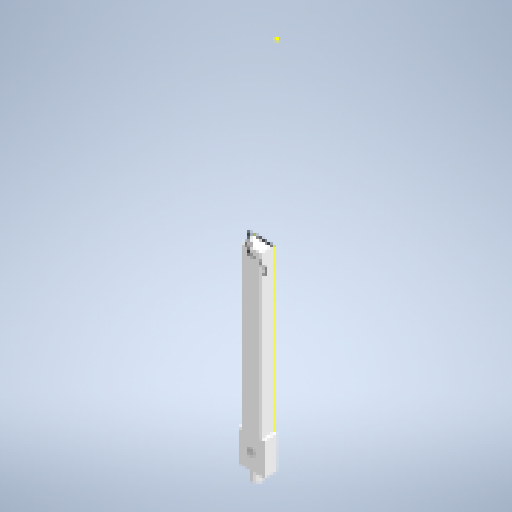
# Autodesk Inventor part: SchubstangeA
Saved by Autodesk Inventor 2025 (Build 290162010, 162A)
## iProperties
Created: 2024-11-26
Part Number: SchubstangeA
Material: PC/ABS-Kunststoff, 3DDruck, PLA
Document SubType Name: Modeling
Designer: Admin
Density: 1.1 g/cm^3
Appearance: Glatt - Weiß(2)
Author: Admin
Autodesk Inventor part; units mm, degrees
ref_plane "YZ Plane" through (0, 0, 0) normal (1, 0, 0) x (0, 1, 0)
ref_plane "XZ Plane" through (0, 0, 0) normal (0, 1, 0) x (-1, 0, 0)
ref_plane "XY Plane" through (0, 0, 0) normal (0, 0, 1) x (1, 0, 0)
sketch "Skizze1" plane through (0, 0, 0) normal (0, 1, 0) x (-1, 0, 0)
  line L0 (6.8592, -116.2444) -> (0.8592, -116.2444)
  line L1 (0.8592, -116.2444) -> (0.8592, -56.2444)
  line L2 (6.8592, -56.2444) -> (6.8592, -116.2444)
  line L3 (7.8592, -116.2444) -> (-0.1408, -116.2444)
  line L4 (-0.1408, -116.2444) -> (-0.1408, -106.2444)
  line L5 (-0.1408, -106.2444) -> (7.8592, -106.2444)
  line L6 (7.8592, -106.2444) -> (7.8592, -116.2444)
  line L7 (3.8592, 157.3916) -> (3.8592, -262.6084)
  line L8 (6.8592, -56.2444) -> (0.8592, -56.2444)
  line L9 (0.8592, -56.2444) -> (-2.1408, -56.2444)
  line L10 (-2.1408, -56.2444) -> (-2.1408, -66.2444)
  line L11 (-2.1408, -66.2444) -> (0.8592, -66.2444)
  line L12 (0.8592, -66.2444) -> (0.8592, -56.2444)
  line L13 (6.8592, -56.2444) -> (9.8592, -56.2444)
  line L14 (9.8592, -56.2444) -> (9.8592, -66.2444)
  line L15 (9.8592, -66.2444) -> (6.8592, -66.2444)
  line L16 (6.8592, -66.2444) -> (6.8592, -56.2444)
  point P0 (0, 0)
  point P1 (0.8592, -106.2444)
  point P2 (6.8592, -106.2444)
  point P3 (6.8592, -116.2444)
  point P4 (3.8592, -116.2444)
  point P5 (6.8592, -66.2444)
  point P6 (0.8592, -66.2444)
  dimension "d1" = 60
  dimension "d9" = 6
  dimension "d25" = 8
  dimension "d26" = 10
  dimension "d27" = 1
  dimension "d44" = 3
  dimension "d45" = 10
  dimension "d46" = 3
  constraints: 34 end point, 7 parallel, 6 horizontal, 4 perpendicular, 2 point on line, 1 collinear, 1 midpoint, 1 vertical, 2 other
  measures "d1" distance of L0.end L1.end
  measures "d9" distance of L0.start L0.end
  measures "d25" distance of L4.end L5.end
  measures "d26" distance of L3.end L4.end
  measures "d27" distance of L3.end L0.end
  measures "d44" distance of L11.end L10.end
  measures "d45" distance of L10.end L9.end
  measures "d46" distance of L14.end L15.end
extrude "Extrusion1" add sketch "Skizze1" along normal blind 4
sketch "Skizze2" plane through (0, 4, 0) normal (0, 1, 0) x (1, 0, 0)
  line L0 (-3.8592, 111.2444) -> (-6.8592, 111.2444) construction
  line L1 (-3.8592, 111.2444) -> (-0.8592, 111.2444) construction
  line L2 (-0.8592, 66.2444) -> (-0.8592, 106.2444) construction
  line L3 (-6.8592, 106.2444) -> (-6.8592, 66.2444) construction
  line L4 (0.1408, 116.2444) -> (-7.8592, 116.2444) projected
  point P0 (0, 0)
  point P1 (-0.8592, 56.2444)
  point P2 (-6.8592, 56.2444)
  point P3 (-0.8592, 16.2444)
  point P4 (-6.8592, 16.2444)
  dimension "d28" = 5
  constraints: 4 end point, 2 horizontal, 2 point on line, 1 collinear
  measures "d28" distance from line of L4 L0.start
hole "Bohrung1" at (-3.8592, 4, -111.2444) direction (0, -1, 0) diameter 2.459 end through all thread size "M3x0.5" class "6H" standard "ANSI Metric M Profile"
sketch "Skizze3" plane through (0.1408, 0, -116.2444) normal (0, 0, -1) x (-1, 0, 0)
  line L0 (4, 0) -> (4, 1.7)
  circle A0 centre (4, 1.7) radius 1.5
  line L1 (0, 0) -> (8, 0) projected
  point P0 (0.1408, 0)
  dimension "d29" = 3
  dimension "d30" = 1.7
  constraints: 3 end point, 1 centre point, 1 midpoint, 1 perpendicular
  measures "d29" diameter of A0
  measures "d30" distance from line of L1 L0.end
extrude "Extrusion2" add sketch "Skizze3" along normal blind 3
sketch "Skizze5" plane through (0, 4, 0) normal (0, 1, 0) x (1, 0, 0)
  line L0 (2.1408, 56.2444) -> (-9.8592, 56.2444)
  line L1 (-9.8592, 66.2444) -> (2.1408, 66.2444)
  line L2 (2.1408, 66.2444) -> (2.1408, 56.2444)
  line L3 (-5.3592, 56.2444) -> (-2.3592, 56.2444)
  line L4 (-2.3592, 56.2444) -> (-2.3592, 66.2444)
  line L5 (-2.3592, 66.2444) -> (-5.3592, 66.2444)
  line L6 (-5.3592, 66.2444) -> (-5.3592, 56.2444)
  line L7 (-5.3592, 61.2444) -> (-9.8592, 61.2444) construction
  line L8 (-2.3592, 61.2444) -> (2.1408, 61.2444) construction
  line L9 (-9.8592, 66.2444) -> (-9.8592, 56.2444)
  point P0 (0, 0)
  point P1 (-2.3592, 56.2444)
  dimension "d43" = 3
  constraints: 20 end point, 4 midpoint, 4 parallel, 3 coincident, 2 horizontal, 2 point on line, 1 collinear, 1 perpendicular, 1 vertical
  measures "d43" distance between parallel lines of L6 L4
extrude "Extrusion4" add sketch "Skizze5" along normal blind 20 contours L0 L4 L1 L2 | L0 L9 L1 L6
